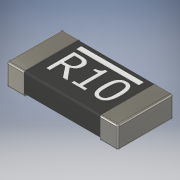
# Autodesk Inventor part: Resistor_1608-0.5mm
Saved by Autodesk Inventor 2018 (Build 220112000, 112)
## iProperties
Created: 2016-08-15
Part Number: Resistor_1608-0.5mm
Material: Copper
Document SubType Name: Modeling
Designer: Bradley
Density: 8.94 g/cm^3
Appearance: Smooth - Black
Author: Bradley
Autodesk Inventor part; units mm, degrees
ref_plane "YZ Plane" through (0, 0, 0) normal (1, 0, 0) x (0, 1, 0)
ref_plane "XZ Plane" through (0, 0, 0) normal (0, 1, 0) x (-1, 0, 0)
ref_plane "XY Plane" through (0, 0, 0) normal (0, 0, 1) x (1, 0, 0)
sketch "Sketch1" plane through (0, 0, 0) normal (0, 0, 1) x (1, 0, 0)
  line L0 (-1.6, 0.585) -> (-1.092, 0.585)
  line L1 (-1.092, 0.585) -> (-1.092, -0.05)
  line L2 (-1.092, -0.05) -> (-1.6, -0.05)
  line L3 (-1.6, -0.05) -> (-1.6, 0.585)
  line L4 (-1.092, 0.575) -> (1.092, 0.575)
  line L5 (1.092, 0.575) -> (1.092, 0)
  line L6 (1.092, 0) -> (-1.092, 0)
  line L7 (-1.092, 0) -> (-1.092, 0.575)
  line L8 (1.092, 0.585) -> (1.6, 0.585)
  line L9 (1.6, 0.585) -> (1.6, -0.05)
  line L10 (1.6, -0.05) -> (1.092, -0.05)
  line L11 (1.092, -0.05) -> (1.092, 0.585)
  point P0 (0, 0)
  point P1 (0, 0.575)
  point P2 (0, 0)
  dimension "d0" = 3.2
  dimension "d1" = 0.635
  dimension "d2" = 0.508
  dimension "d3" = 0.05
  dimension "d6" = 0.01
  constraints: 24 end point, 6 parallel, 3 horizontal, 3 perpendicular, 3 point on line, 2 collinear, 2 midpoint, 1 coincident, 1 vertical alignment
  measures "d0" distance between parallel lines of L9 L3
  measures "d1" distance of L2.end L0.start
  measures "d2" distance of L1.end L2.end
  measures "d3" distance between parallel lines of L2 L6
  measures "d6" distance between parallel lines of L4 L0
extrude "Extrusion1" add sketch "Sketch1" along normal mid plane 1.6 contours L0 L1 L2 L3 | L11 L8 L9 L10 L5
extrude "Extrusion2" add sketch "Sketch1" along normal mid plane 1.59 contours L4 L5 L6 L1
sketch "Sketch3" plane through (-1.092, 0.575, 0.84) normal (0, 1, 0) x (1, 0, 0)
  line L0 (0, 0.045) -> (0, 1.635) projected
  line L1 (2.184, 0.045) -> (0, 0.045) projected
  line L2 (2.184, 1.635) -> (2.184, 0.045) projected
  line L3 (0, 1.635) -> (2.184, 1.635) projected
  line L4 (2.184, 1.64) -> (2.184, 0.04) construction
  line L5 (2.184, 0.84) -> (0, 0.84) construction
  line L6 (0, 1.64) -> (0, 0.04) construction
  line L7 (0.192, 1.49) -> (1.992, 1.49)
  line L8 (1.992, 1.49) -> (1.992, 1.34)
  line L9 (1.992, 1.34) -> (0.192, 1.34)
  line L10 (0.192, 1.34) -> (0.192, 1.49)
  line L11 (0.8505, 0.44) -> (0.7124, 0.44)
  line L12 (0.7124, 0.44) -> (0.4596, 0.7583)
  line L13 (0.4596, 0.7583) -> (0.3377, 0.7583)
  line L14 (0.3377, 0.7583) -> (0.3377, 0.44)
  line L15 (0.3377, 0.44) -> (0.2314, 0.44)
  line L16 (0.2314, 0.44) -> (0.2314, 1.24)
  line L17 (0.2314, 1.24) -> (0.4375, 1.24)
  spline S0 degree 2 poles (0.4375, 1.24) (0.5063, 1.24) (0.599, 1.2251) (0.6411, 1.1979) knots 0 0 0 1 2 2 2
  spline S1 degree 2 poles (0.6411, 1.1979) (0.6832, 1.1706) (0.7319, 1.0857) (0.7319, 1.0228) knots 0 0 0 1 2 2 2
  spline S2 degree 2 poles (0.7319, 1.0228) (0.7319, 0.9353) (0.6424, 0.8167) (0.5659, 0.7881) knots 0 0 0 1 2 2 2
  line L18 (0.5659, 0.7881) -> (0.8505, 0.44)
  spline S3 degree 2 poles (0.621, 1.0144) (0.621, 1.0494) (0.5964, 1.1032) (0.5704, 1.1207) knots 0 0 0 1 2 2 2
  spline S4 degree 2 poles (0.5704, 1.1207) (0.5478, 1.1356) (0.4875, 1.1479) (0.4434, 1.1479) knots 0 0 0 1 2 2 2
  line L19 (0.4434, 1.1479) -> (0.3377, 1.1479)
  line L20 (0.3377, 1.1479) -> (0.3377, 0.8471)
  line L21 (0.3377, 0.8471) -> (0.4311, 0.8471)
  spline S5 degree 2 poles (0.4311, 0.8471) (0.4771, 0.8471) (0.5503, 0.8633) (0.5756, 0.8886) knots 0 0 0 1 2 2 2
  spline S6 degree 2 poles (0.5756, 0.8886) (0.599, 0.9107) (0.621, 0.9729) (0.621, 1.0144) knots 0 0 0 1 2 2 2
  line L22 (1.3445, 0.44) -> (0.9542, 0.44)
  line L23 (0.9542, 0.44) -> (0.9542, 0.5217)
  line L24 (0.9542, 0.5217) -> (1.0995, 0.5217)
  line L25 (1.0995, 0.5217) -> (1.0995, 1.0578)
  line L26 (1.0995, 1.0578) -> (0.9542, 1.0578)
  line L27 (0.9542, 1.0578) -> (0.9542, 1.1311)
  spline S7 degree 2 poles (0.9542, 1.1311) (1.0366, 1.1311) (1.1144, 1.1778) (1.1196, 1.2426) knots 0 0 0 1 2 2 2
  line L28 (1.1196, 1.2426) -> (1.2025, 1.2426)
  line L29 (1.2025, 1.2426) -> (1.2025, 0.5217)
  line L30 (1.2025, 0.5217) -> (1.3445, 0.5217)
  line L31 (1.3445, 0.5217) -> (1.3445, 0.44)
  spline S8 degree 2 poles (1.9896, 0.84) (1.9896, 0.6248) (1.8644, 0.4231) (1.7341, 0.4231) knots 0 0 0 1 2 2 2
  spline S9 degree 2 poles (1.7341, 0.4231) (1.6019, 0.4231) (1.4781, 0.6287) (1.4781, 0.8394) knots 0 0 0 1 2 2 2
  spline S10 degree 2 poles (1.4781, 0.8394) (1.4781, 1.0559) (1.6032, 1.2562) (1.7341, 1.2562) knots 0 0 0 1 2 2 2
  spline S11 degree 2 poles (1.7341, 1.2562) (1.8657, 1.2562) (1.9896, 1.0488) (1.9896, 0.84) knots 0 0 0 1 2 2 2
  spline S12 degree 2 poles (1.8521, 0.5962) (1.8677, 0.6358) (1.8807, 0.7577) (1.8807, 0.84) knots 0 0 0 1 2 2 2
  spline S13 degree 2 poles (1.8807, 0.84) (1.8807, 0.9223) (1.8677, 1.0436) (1.8515, 1.0844) knots 0 0 0 1 2 2 2
  spline S14 degree 2 poles (1.8515, 1.0844) (1.8353, 1.1253) (1.7789, 1.1674) (1.7341, 1.1674) knots 0 0 0 1 2 2 2
  spline S15 degree 2 poles (1.7341, 1.1674) (1.6894, 1.1674) (1.6317, 1.1253) (1.6149, 1.0831) knots 0 0 0 1 2 2 2
  spline S16 degree 2 poles (1.6149, 1.0831) (1.5986, 1.0423) (1.587, 0.9178) (1.587, 0.8394) knots 0 0 0 1 2 2 2
  spline S17 degree 2 poles (1.587, 0.8394) (1.587, 0.7551) (1.5973, 0.6423) (1.6142, 0.5982) knots 0 0 0 1 2 2 2
  spline S18 degree 2 poles (1.6142, 0.5982) (1.6298, 0.5567) (1.6875, 0.512) (1.7341, 0.512) knots 0 0 0 1 2 2 2
  spline S19 degree 2 poles (1.7341, 0.512) (1.7782, 0.512) (1.8359, 0.5541) (1.8521, 0.5962) knots 0 0 0 1 2 2 2
  point P0 (1.092, 0.84)
  point P1 (1.092, 1.34)
  point P2 (1.092, 0.84)
  dimension "d15" = 0.15
  dimension "d16" = 1.8
  dimension "d17" = 0.5
  constraints: 10 end point, 5 midpoint, 2 horizontal, 2 parallel, 2 perpendicular, 1 vertical alignment
  measures "d15" distance of L9.end L7.start
  measures "d16" distance of L7.start L7.end
  measures "d17" distance between parallel lines of L5 L9
extrude "Extrusion4" add sketch "Sketch3" along normal blind 0.01 contours L7 L8 L9 L10 | L11 L12 L13 L14 L15 L16 L17 S0 S1 S2 L18 | L22 L23 L24 L25 L26 L27 S7 L28 L29 L30 L31 | S8 S9 S10 S11
fillet "Fillet2" radius 0.05 4 edges at (0, 0.575, 0.795) (0, 0, 0.795) (0, 0.575, -0.795) (0, 0, -0.795)
fillet "Fillet1" radius 0.05 16 edges at (-1.346, 0.585, 0.8) (1.346, 0.585, 0.8) (-1.346, 0.585, -0.8) (1.346, 0.585, -0.8) (1.6, 0.585, 0) (1.6, 0.2675, -0.8) (1.6, -0.05, 0) (1.346, -0.05, -0.8) (1.346, -0.05, 0.8) (1.6, 0.2675, 0.8) (-1.346, -0.05, -0.8) (-1.6, -0.05, 0) (-1.6, 0.2675, 0.8) (-1.346, -0.05, 0.8) (-1.6, 0.2675, -0.8) (-1.6, 0.585, 0)
body "Solid1"
